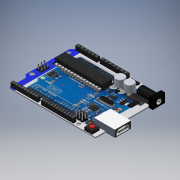
# Autodesk Inventor part: ardino
Saved by Autodesk Inventor 2019 (Build 230136000, 136)
## iProperties
Created: 2020-12-08
Part Number: ardino
Material: Aluminum 6061-AHC
Document SubType Name: Modeling
Designer: 2019u
Density: 2.7 g/cm^3
Appearance: Aluminum - Polished
Author: 2019u
Autodesk Inventor part; units mm, degrees
ref_plane "YZ Plane" through (0, 0, 0) normal (1, 0, 0) x (0, 1, 0)
ref_plane "XZ Plane" through (0, 0, 0) normal (0, 1, 0) x (-1, 0, 0)
ref_plane "XY Plane" through (0, 0, 0) normal (0, 0, 1) x (1, 0, 0)
sketch "Sketch1" plane through (0, 0, 0) normal (0, 1, 0) x (-1, 0, 0)
  line L0 (0, 0) -> (99.3908, 0) construction
  line L1 (99.3908, 0) -> (99.3908, -99.3908) construction
  line L2 (99.3908, -99.3908) -> (0, -99.3908) construction
  line L3 (0, -99.3908) -> (0, 0) construction
  line L4 (94.1362, -15.3552) -> (10.2114, -15.3552)
  line L5 (10.2114, -15.3552) -> (10.2114, -25.1728)
  line L6 (10.2114, -25.1728) -> (0, -25.1728)
  line L7 (1.1362, -25.1728) -> (1.1362, -40.953)
  line L8 (1.1362, -40.953) -> (10.2114, -40.953)
  line L9 (10.2114, -40.953) -> (10.2114, -67.1342)
  line L10 (10.2114, -67.1342) -> (8.5885, -67.1342)
  line L11 (6.3655, -68.1381) -> (6.3655, -79.1042)
  line L12 (8.5885, -79.5442) -> (10.2114, -79.5442)
  line L13 (10.2114, -79.5442) -> (10.2114, -83.1265)
  line L14 (10.2114, -83.1265) -> (94.9443, -83.1265)
  line L15 (94.9443, -83.1265) -> (94.9443, -80.9195)
  line L16 (94.9443, -80.9195) -> (97.9355, -77.6084)
  line L17 (97.9355, -77.6084) -> (98.096, -34.4505)
  line L18 (98.096, -34.4505) -> (94.9443, -31.6032)
  line L19 (94.9443, -31.6032) -> (95.0011, -16.3408)
  arc A0 (95.0011, -16.3408) -> (94.1362, -15.3552) centre (93.5899, -16.7068) ccw
  line L20 (10.2114, -25.1728) -> (21.2581, -25.1728)
  line L21 (21.2581, -25.1728) -> (21.2581, -40.953)
  line L22 (21.2581, -40.953) -> (10.2114, -40.953)
  line L23 (10.2114, -67.1342) -> (10.2114, -68.0566)
  line L24 (10.2114, -79.1042) -> (10.2114, -79.5442)
  line L25 (94.5949, -16.4252) -> (68.0366, -16.4252)
  line L26 (68.0366, -16.4252) -> (68.0366, -19.2086)
  line L27 (68.0366, -19.2086) -> (94.5949, -19.2086)
  line L28 (94.5949, -19.2086) -> (94.5949, -16.4252)
  line L29 (64.6828, -16.0728) -> (32.7155, -16.0728)
  line L30 (32.7155, -16.0728) -> (32.7155, -18.833)
  line L31 (32.7155, -18.833) -> (64.6828, -18.833)
  line L32 (64.6828, -18.833) -> (64.6828, -16.0728)
  line L33 (92.7813, -58.1151) -> (46.6733, -58.1151)
  line L34 (46.6733, -58.1151) -> (46.6733, -67.7931)
  line L35 (46.6733, -67.7931) -> (92.7813, -67.7931)
  line L36 (92.7813, -67.7931) -> (92.7813, -58.1151)
  line L37 (38.3786, -36.2645) -> (32.5411, -36.2645)
  line L38 (32.5411, -36.2645) -> (32.5411, -41.7109)
  line L39 (32.5411, -41.7109) -> (38.3786, -41.7109)
  line L40 (38.3786, -41.7109) -> (38.3786, -36.2645)
  line L41 (38.0929, -47.7922) -> (29.7352, -47.7922)
  line L42 (29.7352, -47.7922) -> (29.7352, -52.5671)
  line L43 (29.7352, -52.5671) -> (38.0929, -52.5671)
  line L44 (38.0929, -52.5671) -> (38.0929, -47.7922)
  arc A1 (38.0929, -52.5671) -> (38.0929, -47.7922) centre (38.0929, -50.1797) ccw
  arc A2 (29.7352, -47.7922) -> (29.7352, -52.5671) centre (29.7352, -50.1797) ccw
  circle A3 centre (42.8477, -72.0836) radius 4.3989
  circle A4 centre (33.5477, -72.0836) radius 4.3076
  line L45 (36.2266, -55.7996) -> (32.5411, -55.7996)
  line L46 (32.5411, -55.7996) -> (32.5411, -59.4796)
  line L47 (32.5411, -59.4796) -> (36.2266, -59.4796)
  line L48 (36.2266, -59.4796) -> (36.2266, -55.7996)
  line L49 (94.1362, -79.3242) -> (72.919, -79.3242)
  line L50 (72.919, -79.3242) -> (72.919, -82.3228)
  line L51 (72.919, -82.3228) -> (94.1362, -82.3228)
  line L52 (94.1362, -82.3228) -> (94.1362, -79.3242)
  line L53 (70.678, -79.9168) -> (44.0674, -79.9168)
  line L54 (44.0674, -79.9168) -> (44.0674, -82.6646)
  line L55 (44.0674, -82.6646) -> (70.678, -82.6646)
  line L56 (70.678, -82.6646) -> (70.678, -79.9168)
  line L57 (41.6475, -79.3242) -> (33.5477, -79.3242)
  line L58 (33.5477, -79.3242) -> (33.5477, -82.3228)
  line L59 (33.5477, -82.3228) -> (41.6475, -82.3228)
  line L60 (41.6475, -82.3228) -> (41.6475, -79.3242)
  line L61 (91.1629, -43.127) -> (96.9206, -43.127)
  line L62 (96.9206, -43.127) -> (96.9206, -52.2064)
  line L63 (96.9206, -52.2064) -> (91.1629, -52.2064)
  line L64 (91.1629, -52.2064) -> (91.1629, -43.127)
  line L65 (10.2114, -68.0566) -> (10.2114, -79.1042)
  line L66 (10.2114, -78.709) -> (10.2114, -67.1342)
  line L67 (10.2114, -79.1042) -> (10.2114, -79.5442)
  line L68 (10.2114, -79.5442) -> (6.3655, -79.5442)
  line L69 (6.3655, -79.5442) -> (6.3655, -67.5295)
  line L70 (6.3655, -67.5295) -> (10.2114, -67.5295)
  line L71 (10.2114, -67.5295) -> (10.2114, -79.5442)
  line L72 (10.2114, -78.0442) -> (24.0286, -78.0442)
  line L73 (24.0286, -78.0442) -> (24.0286, -69.0295)
  line L74 (24.0286, -69.0295) -> (10.2114, -69.0295)
  line L75 (10.2114, -69.0295) -> (10.2114, -78.0442)
  circle A5 centre (17.5453, -19.2086) radius 2.0145
  line L76 (14.0816, -23.069) -> (21.6028, -23.069)
  line L77 (21.6028, -23.069) -> (21.6028, -15.7452)
  line L78 (21.6028, -15.7452) -> (14.0816, -15.7452)
  line L79 (14.0816, -15.7452) -> (14.0816, -23.069)
  line L80 (28.7929, -26.9178) -> (37.8553, -26.9178)
  line L81 (37.8553, -26.9178) -> (37.8553, -20.8454)
  line L82 (37.8553, -20.8454) -> (28.7929, -20.8454)
  line L83 (28.7929, -20.8454) -> (28.7929, -26.9178)
  line L84 (29.24, -26.4718) -> (31.1601, -26.4718)
  line L85 (31.1601, -26.4718) -> (31.1601, -24.2418)
  line L86 (31.1601, -24.2418) -> (29.24, -24.2418)
  line L87 (29.24, -24.2418) -> (29.24, -26.4718)
  line L88 (32.24, -24.2418) -> (32.24, -26.4718)
  line L89 (34.1601, -26.4718) -> (34.1601, -24.2418)
  line L90 (32.24, -26.4718) -> (34.1601, -26.4718)
  line L91 (34.1601, -24.2418) -> (32.24, -24.2418)
  line L92 (35.24, -24.2418) -> (35.24, -26.4718)
  line L93 (37.1601, -26.4718) -> (37.1601, -24.2418)
  line L94 (35.24, -26.4718) -> (37.1601, -26.4718)
  line L95 (37.1601, -24.2418) -> (35.24, -24.2418)
  line L96 (29.24, -21.2418) -> (29.24, -23.4718)
  line L97 (31.1601, -23.4718) -> (31.1601, -21.2418)
  line L98 (29.24, -23.4718) -> (31.1601, -23.4718)
  line L99 (31.1601, -21.2418) -> (29.24, -21.2418)
  line L100 (32.24, -21.2418) -> (32.24, -23.4718)
  line L101 (34.1601, -23.4718) -> (34.1601, -21.2418)
  line L102 (32.24, -23.4718) -> (34.1601, -23.4718)
  line L103 (34.1601, -21.2418) -> (32.24, -21.2418)
  line L104 (35.24, -21.2418) -> (35.24, -23.4718)
  line L105 (37.1601, -23.4718) -> (37.1601, -21.2418)
  line L106 (35.24, -23.4718) -> (37.1601, -23.4718)
  line L107 (37.1601, -21.2418) -> (35.24, -21.2418)
  circle A6 centre (30.2001, -25.3568) radius 0.4649
  circle A7 centre (33.2001, -25.3568) radius 0.4846
  circle A8 centre (36.2001, -25.3568) radius 0.4567
  circle A9 centre (30.119, -22.3568) radius 0.4825
  circle A10 centre (33.2001, -22.3568) radius 0.4846
  circle A11 centre (36.2001, -22.3568) radius 0.4846
  line L108 (91.1629, -49.1995) -> (100.2253, -49.1995)
  line L109 (100.2253, -49.1995) -> (100.2253, -43.127)
  line L110 (100.2253, -43.127) -> (91.1629, -43.127)
  line L111 (91.1629, -43.127) -> (91.1629, -49.1995)
  line L112 (91.61, -48.7535) -> (93.5302, -48.7535)
  line L113 (93.5302, -48.7535) -> (93.5302, -46.5235)
  line L114 (93.5302, -46.5235) -> (91.61, -46.5235)
  line L115 (91.61, -46.5235) -> (91.61, -48.7535)
  line L116 (94.61, -46.5235) -> (94.61, -48.7535)
  line L117 (96.5302, -48.7535) -> (96.5302, -46.5235)
  line L118 (94.61, -48.7535) -> (96.5302, -48.7535)
  line L119 (96.5302, -46.5235) -> (94.61, -46.5235)
  line L120 (97.61, -46.5235) -> (97.61, -48.7535)
  line L121 (99.5302, -48.7535) -> (99.5302, -46.5235)
  line L122 (97.61, -48.7535) -> (99.5302, -48.7535)
  line L123 (99.5302, -46.5235) -> (97.61, -46.5235)
  line L124 (91.61, -43.5235) -> (91.61, -45.7535)
  line L125 (93.5302, -45.7535) -> (93.5302, -43.5235)
  line L126 (91.61, -45.7535) -> (93.5302, -45.7535)
  line L127 (93.5302, -43.5235) -> (91.61, -43.5235)
  line L128 (94.61, -43.5235) -> (94.61, -45.7535)
  line L129 (96.5302, -45.7535) -> (96.5302, -43.5235)
  line L130 (94.61, -45.7535) -> (96.5302, -45.7535)
  line L131 (96.5302, -43.5235) -> (94.61, -43.5235)
  line L132 (97.61, -43.5235) -> (97.61, -45.7535)
  line L133 (99.5302, -45.7535) -> (99.5302, -43.5235)
  line L134 (97.61, -45.7535) -> (99.5302, -45.7535)
  line L135 (99.5302, -43.5235) -> (97.61, -43.5235)
  circle A12 centre (92.5701, -47.6385) radius 0.4649
  circle A13 centre (95.5701, -47.6385) radius 0.4846
  circle A14 centre (98.5701, -47.6385) radius 0.4567
  circle A15 centre (92.489, -44.6385) radius 0.4825
  circle A16 centre (95.5701, -44.6385) radius 0.4846
  circle A17 centre (98.5701, -44.6385) radius 0.4846
  line L136 (94.61, -51.6653) -> (96.5302, -51.6653)
  circle A18 centre (95.5701, -50.5503) radius 0.4846
  line L137 (94.61, -49.4353) -> (94.61, -51.6653)
  line L138 (96.5302, -51.6653) -> (96.5302, -49.4353)
  line L139 (96.5302, -49.4353) -> (94.61, -49.4353)
  line L140 (97.61, -49.4353) -> (97.61, -51.6653)
  line L141 (91.61, -51.6653) -> (93.5302, -51.6653)
  circle A19 centre (92.5701, -50.5503) radius 0.4649
  line L142 (91.61, -49.4353) -> (91.61, -51.6653)
  line L143 (93.5302, -51.6653) -> (93.5302, -49.4353)
  line L144 (93.5302, -49.4353) -> (91.61, -49.4353)
  line L145 (17.5453, -65.908) -> (21.2581, -65.908)
  line L146 (21.2581, -65.908) -> (21.2581, -57.6396)
  line L147 (21.2581, -57.6396) -> (17.5453, -57.6396)
  line L148 (17.5453, -57.6396) -> (17.5453, -65.908)
  line L149 (37.1601, -66.1422) -> (38.7457, -66.1422)
  line L150 (38.7457, -66.1422) -> (38.7457, -62.7647)
  line L151 (38.7457, -62.7647) -> (37.1601, -62.7647)
  line L152 (37.1601, -62.7647) -> (37.1601, -66.1422)
  line L153 (47.2465, -58.1151) -> (49.4015, -58.1151)
  line L154 (49.4015, -58.1151) -> (49.4015, -56.2579)
  line L155 (49.4015, -56.2579) -> (47.2465, -56.2579)
  line L156 (47.2465, -56.2579) -> (47.2465, -58.1151)
  line L157 (50.2465, -56.2579) -> (50.2465, -58.1151)
  line L158 (52.4015, -56.2579) -> (50.2465, -56.2579)
  line L159 (52.4015, -58.1151) -> (52.4015, -56.2579)
  line L160 (50.2465, -58.1151) -> (52.4015, -58.1151)
  line L161 (53.2465, -56.2579) -> (53.2465, -58.1151)
  line L162 (55.4015, -56.2579) -> (53.2465, -56.2579)
  line L163 (55.4015, -58.1151) -> (55.4015, -56.2579)
  line L164 (53.2465, -58.1151) -> (55.4015, -58.1151)
  line L165 (56.2465, -56.2579) -> (56.2465, -58.1151)
  line L166 (58.4015, -56.2579) -> (56.2465, -56.2579)
  line L167 (58.4015, -58.1151) -> (58.4015, -56.2579)
  line L168 (56.2465, -58.1151) -> (58.4015, -58.1151)
  line L169 (59.2465, -56.2579) -> (59.2465, -58.1151)
  line L170 (61.4015, -56.2579) -> (59.2465, -56.2579)
  line L171 (61.4015, -58.1151) -> (61.4015, -56.2579)
  line L172 (59.2465, -58.1151) -> (61.4015, -58.1151)
  line L173 (62.2465, -56.2579) -> (62.2465, -58.1151)
  line L174 (64.4015, -56.2579) -> (62.2465, -56.2579)
  line L175 (64.4015, -58.1151) -> (64.4015, -56.2579)
  line L176 (62.2465, -58.1151) -> (64.4015, -58.1151)
  line L177 (65.2465, -56.2579) -> (65.2465, -58.1151)
  line L178 (67.4015, -56.2579) -> (65.2465, -56.2579)
  line L179 (67.4015, -58.1151) -> (67.4015, -56.2579)
  line L180 (65.2465, -58.1151) -> (67.4015, -58.1151)
  line L181 (68.2465, -56.2579) -> (68.2465, -58.1151)
  line L182 (70.4015, -56.2579) -> (68.2465, -56.2579)
  line L183 (70.4015, -58.1151) -> (70.4015, -56.2579)
  line L184 (68.2465, -58.1151) -> (70.4015, -58.1151)
  line L185 (71.2465, -56.2579) -> (71.2465, -58.1151)
  line L186 (73.4015, -56.2579) -> (71.2465, -56.2579)
  line L187 (73.4015, -58.1151) -> (73.4015, -56.2579)
  line L188 (71.2465, -58.1151) -> (73.4015, -58.1151)
  line L189 (74.2465, -56.2579) -> (74.2465, -58.1151)
  line L190 (76.4015, -56.2579) -> (74.2465, -56.2579)
  line L191 (76.4015, -58.1151) -> (76.4015, -56.2579)
  line L192 (74.2465, -58.1151) -> (76.4015, -58.1151)
  line L193 (77.2465, -56.2579) -> (77.2465, -58.1151)
  line L194 (79.4015, -56.2579) -> (77.2465, -56.2579)
  line L195 (79.4015, -58.1151) -> (79.4015, -56.2579)
  line L196 (77.2465, -58.1151) -> (79.4015, -58.1151)
  line L197 (80.2465, -56.2579) -> (80.2465, -58.1151)
  line L198 (82.4015, -56.2579) -> (80.2465, -56.2579)
  line L199 (82.4015, -58.1151) -> (82.4015, -56.2579)
  line L200 (80.2465, -58.1151) -> (82.4015, -58.1151)
  line L201 (83.2465, -56.2579) -> (83.2465, -58.1151)
  line L202 (85.4015, -56.2579) -> (83.2465, -56.2579)
  line L203 (85.4015, -58.1151) -> (85.4015, -56.2579)
  line L204 (83.2465, -58.1151) -> (85.4015, -58.1151)
  line L205 (86.2465, -56.2579) -> (86.2465, -58.1151)
  line L206 (88.4015, -56.2579) -> (86.2465, -56.2579)
  line L207 (88.4015, -58.1151) -> (88.4015, -56.2579)
  line L208 (86.2465, -58.1151) -> (88.4015, -58.1151)
  line L209 (89.2465, -56.2579) -> (89.2465, -58.1151)
  line L210 (91.4015, -56.2579) -> (89.2465, -56.2579)
  line L211 (91.4015, -58.1151) -> (91.4015, -56.2579)
  line L212 (89.2465, -58.1151) -> (91.4015, -58.1151)
  line L213 (47.2465, -67.7747) -> (47.2465, -69.6318)
  line L214 (49.4015, -67.7747) -> (47.2465, -67.7747)
  line L215 (49.4015, -69.6318) -> (49.4015, -67.7747)
  line L216 (47.2465, -69.6318) -> (49.4015, -69.6318)
  line L217 (50.2465, -67.7747) -> (50.2465, -69.6318)
  line L218 (52.4015, -67.7747) -> (50.2465, -67.7747)
  line L219 (52.4015, -69.6318) -> (52.4015, -67.7747)
  line L220 (50.2465, -69.6318) -> (52.4015, -69.6318)
  line L221 (53.2465, -67.7747) -> (53.2465, -69.6318)
  line L222 (55.4015, -67.7747) -> (53.2465, -67.7747)
  line L223 (55.4015, -69.6318) -> (55.4015, -67.7747)
  line L224 (53.2465, -69.6318) -> (55.4015, -69.6318)
  line L225 (56.2465, -67.7747) -> (56.2465, -69.6318)
  line L226 (58.4015, -67.7747) -> (56.2465, -67.7747)
  line L227 (58.4015, -69.6318) -> (58.4015, -67.7747)
  line L228 (56.2465, -69.6318) -> (58.4015, -69.6318)
  line L229 (59.2465, -67.7747) -> (59.2465, -69.6318)
  line L230 (61.4015, -67.7747) -> (59.2465, -67.7747)
  line L231 (61.4015, -69.6318) -> (61.4015, -67.7747)
  line L232 (59.2465, -69.6318) -> (61.4015, -69.6318)
  line L233 (62.2465, -67.7747) -> (62.2465, -69.6318)
  line L234 (64.4015, -67.7747) -> (62.2465, -67.7747)
  line L235 (64.4015, -69.6318) -> (64.4015, -67.7747)
  line L236 (62.2465, -69.6318) -> (64.4015, -69.6318)
  line L237 (65.2465, -67.7747) -> (65.2465, -69.6318)
  line L238 (67.4015, -67.7747) -> (65.2465, -67.7747)
  line L239 (67.4015, -69.6318) -> (67.4015, -67.7747)
  line L240 (65.2465, -69.6318) -> (67.4015, -69.6318)
  line L241 (68.2465, -67.7747) -> (68.2465, -69.6318)
  line L242 (70.4015, -67.7747) -> (68.2465, -67.7747)
  line L243 (70.4015, -69.6318) -> (70.4015, -67.7747)
  line L244 (68.2465, -69.6318) -> (70.4015, -69.6318)
  line L245 (71.2465, -67.7747) -> (71.2465, -69.6318)
  line L246 (73.4015, -67.7747) -> (71.2465, -67.7747)
  line L247 (73.4015, -69.6318) -> (73.4015, -67.7747)
  line L248 (71.2465, -69.6318) -> (73.4015, -69.6318)
  line L249 (74.2465, -67.7747) -> (74.2465, -69.6318)
  line L250 (76.4015, -67.7747) -> (74.2465, -67.7747)
  line L251 (76.4015, -69.6318) -> (76.4015, -67.7747)
  line L252 (74.2465, -69.6318) -> (76.4015, -69.6318)
  line L253 (77.2465, -67.7747) -> (77.2465, -69.6318)
  line L254 (79.4015, -67.7747) -> (77.2465, -67.7747)
  line L255 (79.4015, -69.6318) -> (79.4015, -67.7747)
  line L256 (77.2465, -69.6318) -> (79.4015, -69.6318)
  line L257 (80.2465, -67.7747) -> (80.2465, -69.6318)
  line L258 (82.4015, -67.7747) -> (80.2465, -67.7747)
  line L259 (82.4015, -69.6318) -> (82.4015, -67.7747)
  line L260 (80.2465, -69.6318) -> (82.4015, -69.6318)
  line L261 (83.2465, -67.7747) -> (83.2465, -69.6318)
  line L262 (85.4015, -67.7747) -> (83.2465, -67.7747)
  line L263 (85.4015, -69.6318) -> (85.4015, -67.7747)
  line L264 (83.2465, -69.6318) -> (85.4015, -69.6318)
  line L265 (86.2465, -67.7747) -> (86.2465, -69.6318)
  line L266 (88.4015, -67.7747) -> (86.2465, -67.7747)
  line L267 (88.4015, -69.6318) -> (88.4015, -67.7747)
  line L268 (86.2465, -69.6318) -> (88.4015, -69.6318)
  line L269 (89.2465, -67.7747) -> (89.2465, -69.6318)
  line L270 (91.4015, -67.7747) -> (89.2465, -67.7747)
  line L271 (91.4015, -69.6318) -> (91.4015, -67.7747)
  line L272 (89.2465, -69.6318) -> (91.4015, -69.6318)
  line L273 (93.5302, -56.2579) -> (46.4999, -56.2579)
  line L274 (46.4999, -56.2579) -> (46.4999, -69.6318)
  line L275 (46.4999, -69.6318) -> (93.5302, -69.6318)
  line L276 (93.5302, -69.6318) -> (93.5302, -56.2579)
  dimension "d4" = 9.3
  dimension "d68" = 1.5
  dimension "d69" = 1.5
  dimension "d83" = 3
  dimension "d86" = 3
  dimension "d99" = 3
  dimension "d100" = 3
  dimension "d112" = 3
  dimension "d133" = 3
  dimension "d136" = 11.5168
  dimension "d194" = 99.3908
  constraints: 546 end point, 46 parallel, 32 perpendicular, 27 horizontal, 19 centre point, 12 point on line, 6 point on circle, 5 vertical, 4 tangent, 317 other
  measures "d4" distance of A4.centre point (42.848, -72.084)
  measures "d68" distance between parallel lines of L74 L70
  measures "d69" distance between parallel lines of L72 L68
  measures "d83" distance of L86.end L88.start
  measures "d86" distance of L86.end L96.start
  measures "d99" distance of L115.start L116.start
  measures "d100" distance of L115.start L124.start
  measures "d112" distance of L144.end L139.end
  measures "d133" distance of L155.end L157.start
  measures "d136" distance of L155.end L213.start
  measures "d194" distance of L2.end L1.end
extrude "Extrusion1" add sketch "Sketch1" against normal blind 1 contours A0 L19 L18 L17 L110 L61 L64 L63 L62 L108 L16 L15 L14 L13 L24 L65 L72 L73 L74 L23 L9 L22 L21 L20 L5 L4 | L17 L135 L132 L134 L123 L120 L122 L108 L62 L110 | L17 L134 L132 L135 | L62 L108 L64 L61 | L62 L63 L64 L108 | L17 L122 L120 L123 | L74 L73 L72 L65 | L28 L27 L26 L25 | L32 L31 L30 L29 | L36 L35 L271 L270 L269 L267 L266 L265 L263 L262 L261 L259 L258 L257 L255 L254 L253 L251 L250 L249 L247 L246 L245 L243 L242 L241 L239 L238 L237 L235 L234 L233 L231 L230 L229 L227 L226 L225 L223 L222 L221 L219 L218 L217 L215 L214 L213 L34 L33 | L33 L211 L273 L276 L275 L271 L35 L36 | L33 L209 L210 L211 | L33 L207 L273 L209 | A3 | L271 L272 L269 L35 | L35 L269 L270 L271 | L33 L205 L206 L207 | L269 L275 L267 L35 | L33 L203 L273 L205 | L267 L268 L265 L35 | L35 L265 L266 L267 | L33 L201 L202 L203 | L265 L275 L263 L35 | L33 L199 L273 L201 | L263 L264 L261 L35 | L35 L261 L262 L263 | L33 L197 L198 L199 | L261 L275 L259 L35 | L33 L195 L273 L197 | L259 L260 L257 L35 | L35 L257 L258 L259 | L33 L193 L194 L195 | L257 L275 L255 L35 | L33 L191 L273 L193 | L255 L256 L253 L35 | L35 L253 L254 L255 | L33 L189 L190 L191 | L253 L275 L251 L35 | L33 L187 L273 L189 | L251 L252 L249 L35 | L35 L249 L250 L251 | L33 L185 L186 L187 | L249 L275 L247 L35 | L33 L183 L273 L185 | L247 L248 L245 L35 | L35 L245 L246 L247 | L33 L181 L182 L183 | L245 L275 L243 L35 | L33 L179 L273 L181 | L243 L244 L241 L35 | L35 L241 L242 L243 | L33 L177 L178 L179 | L241 L275 L239 L35 | L33 L175 L273 L177 | L239 L240 L237 L35 | L35 L237 L238 L239 | L33 L173 L174 L175 | L237 L275 L235 L35 | L33 L171 L273 L173 | L235 L236 L233 L35 | L35 L233 L234 L235 | L33 L169 L170 L171 | L233 L275 L231 L35 | L33 L167 L273 L169 | L231 L232 L229 L35 | L35 L229 L230 L231 | L33 L165 L166 L167 | L229 L275 L227 L35 | L33 L163 L273 L165 | L227 L228 L225 L35 | L35 L225 L226 L227 | L33 L161 L162 L163 | L225 L275 L223 L35 | L33 L159 L273 L161 | L223 L224 L221 L35 | L35 L221 L222 L223 | L33 L157 L158 L159 | L221 L275 L219 L35 | L33 L154 L273 L157 | L219 L220 L217 L35 | L35 L217 L218 L219 | L33 L156 L155 L154 | L217 L275 L215 L35 | L33 L34 L35 L213 L275 L274 L273 L156 | L215 L216 L213 L35 | L35 L213 L214 L215 | L40 L39 L38 L37 | L44 L43 L42 L41 | A1 L44 | L42 A2 | A4 | L48 L47 L46 L45 | L52 L51 L50 L49 | L56 L55 L54 L53 | L60 L59 L58 L57 | A5 | L79 L78 L77 L76 | L83 L82 L81 L80 | L87 L86 L85 L84 | L91 L89 L90 L88 | L95 L93 L94 L92 | L99 L97 L98 L96 | L103 L101 L102 L100 | L107 L105 L106 L104 | A6 | A7 | A8 | A9 | A10 | A11 | L115 L114 L113 L112 | L119 L117 L118 L116 | L127 L125 L126 L124 | L131 L129 L130 L128 | A12 | A13 | A15 | A16 | L137 L139 L138 L136 | A18 | L142 L144 L143 L141 | A19 | L148 L147 L146 L145 | L152 L151 L150 L149
extrude "Extrusion2" add sketch "Sketch1" along normal blind 6 and the other way blind 1 contours L20 L21 L22 L8 L7 L6
extrude "Extrusion3" add sketch "Sketch1" along normal blind 7 contours A3 | A4
extrude "Extrusion4" add sketch "Sketch1" along normal blind 5 contours L36 L35 L271 L270 L269 L267 L266 L265 L263 L262 L261 L259 L258 L257 L255 L254 L253 L251 L250 L249 L247 L246 L245 L243 L242 L241 L239 L238 L237 L235 L234 L233 L231 L230 L229 L227 L226 L225 L223 L222 L221 L219 L218 L217 L215 L214 L213 L34 L33 | L35 L269 L270 L271 | L35 L265 L266 L267 | L35 L261 L262 L263 | L35 L257 L258 L259 | L35 L253 L254 L255 | L35 L249 L250 L251 | L35 L245 L246 L247 | L35 L241 L242 L243 | L35 L237 L238 L239 | L35 L233 L234 L235 | L35 L229 L230 L231 | L35 L225 L226 L227 | L35 L221 L222 L223 | L35 L217 L218 L219 | L35 L213 L214 L215
extrude "Extrusion5" add sketch "Sketch1" along normal blind 2 contours L44 L43 L42 L41 | A1 L44 | L42 A2
extrude "Extrusion6" add sketch "Sketch1" along normal blind 0.5 contours L40 L39 L38 L37 | L48 L47 L46 L45
extrude "Extrusion7" add sketch "Sketch1" along normal blind 4 contours L28 L27 L26 L25 | L32 L31 L30 L29 | L52 L51 L50 L49 | L56 L55 L54 L53
extrude "Extrusion10" add sketch "Sketch1" along normal blind 8 and the other way blind 1 contours L23 L65 L24 L12 L68 L69 L11 L70
extrude "Extrusion11" add sketch "Sketch1" along normal blind 8 contours L74 L73 L72 L65
fillet "Fillet2" radius 4.5 2 edges at (-17.12, 8, -78.0442) (-17.12, 8, -69.0295)
extrude "Extrusion12" add sketch "Sketch1" along normal blind 4 contours A5
extrude "Extrusion13" add sketch "Sketch1" along normal blind 3 contours L79 L78 L77 L76
extrude "Extrusion14" add sketch "Sketch1" along normal blind 5 contours A6 | A7 | A8 | A9 | A10 | A11
extrude "Extrusion15" add sketch "Sketch1" along normal blind 1 contours L87 L86 L85 L84 | L91 L89 L90 L88 | L95 L93 L94 L92 | L99 L97 L98 L96 | L103 L101 L102 L100 | L107 L105 L106 L104
fillet "Fillet3" radius 0.4 6 edges at (-29.7352, 5, -25.3568) (-29.6365, 5, -22.3568) (-32.7155, 5, -25.3568) (-35.7434, 5, -25.3568) (-35.7155, 5, -22.3568) (-32.7155, 5, -22.3568)
extrude "Extrusion16" add sketch "Sketch1" along normal blind 5 contours A12 | A13 | A15 | A16 | A18 | A19
extrude "Extrusion17" add sketch "Sketch1" along normal blind 1 contours L115 L114 L113 L112 | L119 L117 L118 L116 | L127 L125 L126 L124 | L131 L129 L130 L128 | L137 L139 L138 L136 | L142 L144 L143 L141
fillet "Fillet4" radius 0.4 30 edges at (-92.0065, 5, -44.6385) (-95.0855, 5, -44.6385) (-92.1052, 5, -47.6385) (-91.61, 1, -47.6385) (-95.0855, 5, -47.6385) (-95.0855, 5, -50.5503) (-92.1052, 5, -50.5503) (-92.5701, 1, -48.7535) (-93.5302, 1, -47.6385) (-92.5701, 1, -46.5235) (-91.61, 1, -44.6385) (-92.5701, 1, -45.7535) (-92.5701, 1, -43.5235) (-93.5302, 1, -44.6385) (-94.61, 1, -44.6385) (-95.5701, 1, -43.5235) (-96.5302, 1, -44.6385) (-95.5701, 1, -45.7535) (-95.5701, 1, -46.5235) (-94.61, 1, -47.6385) (-95.5701, 1, -48.7535) (-96.5302, 1, -47.6385) (-91.61, 1, -50.5503) (-92.5701, 1, -51.6653) (-92.5701, 1, -49.4353) (-93.5302, 1, -50.5503) (-94.61, 1, -50.5503) (-95.5701, 1, -51.6653) (-95.5701, 1, -49.4353) (-96.5302, 1, -50.5503)
extrude "Extrusion18" add sketch "Sketch1" along normal blind 1 contours L60 L59 L58 L57
extrude "Extrusion19" add sketch "Sketch1" along normal blind 1 contours L148 L147 L146 L145 | L152 L151 L150 L149
sketch "Sketch2" plane through (-6.3655, -1, -79.5442) normal (1, 0, 0) x (0, 0, -1)
  circle A0 centre (-5.7758, 4.0263) radius 2.4717
  circle A1 centre (-5.7758, 4.0263) radius 0.5901
  point P0 (-79.5442, 1)
  constraints: 2 centre point, 1 coincident
extrude "Extrusion20" cut sketch "Sketch2" against normal blind 15
sketch "Sketch3" plane through (-1.1362, -1, -40.953) normal (1, 0, 0) x (0, 0, -1)
  line L0 (-11.132, 5.6691) -> (-4.7121, 5.6691)
  line L1 (-1.7121, 2.6691) -> (-1.7121, 0.6321)
  line L2 (-1.7121, 0.6321) -> (-14.132, 0.6321)
  line L3 (-14.132, 0.6321) -> (-14.132, 2.6691)
  arc A0 (-11.132, 5.6691) -> (-14.132, 2.6691) centre (-11.132, 2.6691) ccw
  arc A1 (-1.7121, 2.6691) -> (-4.7121, 5.6691) centre (-4.7121, 2.6691) ccw
  line L4 (-4.7121, 3.9211) -> (-11.132, 3.9211)
  arc A2 (-11.132, 3.9211) -> (-12.384, 2.6691) centre (-11.132, 2.6691) ccw
  line L5 (-12.384, 2.6691) -> (-12.384, 2.3801)
  line L6 (-12.384, 2.3801) -> (-3.4601, 2.3801)
  line L7 (-3.4601, 2.3801) -> (-3.4601, 2.6691)
  arc A3 (-3.4601, 2.6691) -> (-4.7121, 3.9211) centre (-4.7121, 2.6691) ccw
  line L8 (-10.6435, 3.3982) -> (-5.0624, 3.3982)
  line L9 (-5.0624, 3.3982) -> (-5.0624, 2.8158)
  line L10 (-5.0624, 2.8158) -> (-10.6435, 2.8158)
  line L11 (-10.6435, 2.8158) -> (-10.6435, 3.3982)
  line L12 (-10.6435, 2.8158) -> (-10.2916, 2.8158)
  line L13 (-10.2916, 2.8158) -> (-10.2916, 3.107)
  line L14 (-10.2916, 3.107) -> (-10.6435, 3.107)
  line L15 (-10.6435, 3.107) -> (-10.6435, 2.8158)
  line L16 (-9.8886, 2.8158) -> (-9.5394, 2.8158)
  line L17 (-9.5394, 2.8158) -> (-9.5394, 3.107)
  line L18 (-9.5394, 3.107) -> (-9.8886, 3.107)
  line L19 (-9.8886, 3.107) -> (-9.8886, 2.8158)
  line L20 (-9.1148, 3.107) -> (-8.6537, 3.107)
  line L21 (-8.6537, 3.107) -> (-8.6537, 2.8158)
  line L22 (-8.6537, 2.8158) -> (-9.1148, 2.8158)
  line L23 (-9.1148, 2.8158) -> (-9.1148, 3.107)
  line L24 (-8.3261, 3.107) -> (-8.0592, 3.107)
  line L25 (-8.0592, 3.107) -> (-8.0592, 2.8158)
  line L26 (-8.0592, 2.8158) -> (-8.3261, 2.8158)
  line L27 (-8.3261, 2.8158) -> (-8.3261, 3.107)
  line L28 (-7.853, 3.107) -> (-7.7085, 3.107)
  line L29 (-7.7085, 3.107) -> (-7.7085, 2.8158)
  line L30 (-7.7085, 2.8158) -> (-7.853, 2.8158)
  line L31 (-7.853, 2.8158) -> (-7.853, 3.107)
  line L32 (-7.4162, 3.107) -> (-7.1735, 3.107)
  line L33 (-7.1735, 3.107) -> (-7.1735, 2.8158)
  line L34 (-7.1735, 2.8158) -> (-7.4162, 2.8158)
  line L35 (-7.4162, 2.8158) -> (-7.4162, 3.107)
  line L36 (-6.8945, 3.107) -> (-6.6397, 3.107)
  line L37 (-6.6397, 3.107) -> (-6.6397, 2.8158)
  line L38 (-6.6397, 2.8158) -> (-6.8945, 2.8158)
  line L39 (-6.8945, 2.8158) -> (-6.8945, 3.107)
  line L40 (-6.3485, 3.107) -> (-6.0937, 3.107)
  line L41 (-6.0937, 3.107) -> (-6.0937, 2.8158)
  line L42 (-6.0937, 2.8158) -> (-6.3485, 2.8158)
  line L43 (-6.3485, 2.8158) -> (-6.3485, 3.107)
  line L44 (-5.8025, 3.107) -> (-5.5841, 3.107)
  line L45 (-5.5841, 3.107) -> (-5.5841, 2.8158)
  line L46 (-5.5841, 2.8158) -> (-5.8025, 2.8158)
  line L47 (-5.8025, 2.8158) -> (-5.8025, 3.107)
  line L48 (-5.39, 3.107) -> (-5.2444, 3.107)
  line L49 (-5.2444, 3.107) -> (-5.2444, 2.8158)
  line L50 (-5.2444, 2.8158) -> (-5.39, 2.8158)
  line L51 (-5.39, 2.8158) -> (-5.39, 3.107)
  point P0 (-40.953, 1)
  dimension "d128" = 3
  constraints: 102 end point, 25 parallel, 13 horizontal, 13 perpendicular, 9 point on line, 8 point on circle, 4 centre point, 4 tangent, 1 equal radius, 17 other
  measures "d128" radius of A0
extrude "Extrusion21" cut sketch "Sketch3" against normal blind 15 contours L0 A1 L1 L2 L3 A0 | L8 L9 L10 L49 L48 L51 L45 L44 L47 L41 L40 L43 L37 L36 L39 L33 L32 L35 L29 L28 L31 L25 L24 L27 L21 L20 L23 L17 L18 L19 L13 L14 L11
extrude "Extrusion22" add sketch "Sketch1" along normal blind 1.5 contours L33 L156 L155 L154
pattern_linear "Rectangular Pattern1" count 15 spacing 3 along (-1, 0, 0) count 2 spacing 11.54 along (0, 0, -1) of "Extrusion22"
sketch "Sketch4" plane through (-91.4015, 0, -67.7979) normal (-1, 0, 0) x (0, 0, 1)
  line L0 (0.0048, 0) -> (0.0048, 5) projected
  line L1 (0.0048, 0) -> (-0.9952, 0)
  line L2 (-0.9952, 0) -> (-0.9952, 1)
  line L3 (-0.9952, 1) -> (0.0048, 1)
  line L4 (0.0048, 1) -> (0.0048, 0)
  line L5 (9.6828, 0) -> (0.0048, 0) projected
  line L6 (9.6828, 0) -> (10.6828, 0)
  line L7 (10.6828, 0) -> (10.6828, 1)
  line L8 (10.6828, 1) -> (9.6828, 1)
  line L9 (9.6828, 1) -> (9.6828, 0)
  point P0 (67.7979, 0)
  dimension "d148" = 1
  dimension "d149" = 1
  dimension "d150" = 1
  dimension "d151" = 1
  constraints: 16 end point, 4 parallel, 2 horizontal, 2 perpendicular
  measures "d148" distance of L2.end L3.end
  measures "d149" distance of L1.end L2.end
  measures "d150" distance of L8.end L7.end
  measures "d151" distance of L7.end L6.end
extrude "Extrusion23" cut sketch "Sketch4" against normal blind 46
extrude "Extrusion24" add sketch "Sketch1" along normal blind 0.5 contours L33 L211 L273 L276 L275 L271 L35 L36 | L33 L207 L273 L209 | L269 L275 L267 L35 | L33 L203 L273 L205 | L265 L275 L263 L35 | L33 L199 L273 L201 | L261 L275 L259 L35 | L33 L195 L273 L197 | L257 L275 L255 L35 | L33 L191 L273 L193 | L253 L275 L251 L35 | L33 L187 L273 L189 | L249 L275 L247 L35 | L33 L183 L273 L185 | L245 L275 L243 L35 | L33 L179 L273 L181 | L241 L275 L239 L35 | L33 L175 L273 L177 | L237 L275 L235 L35 | L33 L171 L273 L173 | L233 L275 L231 L35 | L33 L167 L273 L169 | L229 L275 L227 L35 | L33 L163 L273 L165 | L225 L275 L223 L35 | L33 L159 L273 L161 | L221 L275 L219 L35 | L33 L154 L273 L157 | L217 L275 L215 L35 | L33 L34 L35 L213 L275 L274 L273 L156
sketch "Sketch5" plane through (0, 4, 0) normal (0, 1, 0) x (1, 0, 0)
  line L0 (-93.7167, 16.8415) -> (-91.8929, 16.8415)
  line L1 (-91.8929, 16.8415) -> (-91.8929, 18.5718)
  line L2 (-91.8929, 18.5718) -> (-93.7167, 18.5718)
  line L3 (-93.7167, 18.5718) -> (-93.7167, 16.8415)
  line L4 (-90.9167, 18.5718) -> (-90.9167, 16.8415)
  line L5 (-90.9167, 16.8415) -> (-89.0929, 16.8415)
  line L6 (-89.0929, 18.5718) -> (-90.9167, 18.5718)
  line L7 (-89.0929, 16.8415) -> (-89.0929, 18.5718)
  line L8 (-88.1167, 18.5718) -> (-88.1167, 16.8415)
  line L9 (-88.1167, 16.8415) -> (-86.2929, 16.8415)
  line L10 (-86.2929, 18.5718) -> (-88.1167, 18.5718)
  line L11 (-86.2929, 16.8415) -> (-86.2929, 18.5718)
  line L12 (-85.3167, 18.5718) -> (-85.3167, 16.8415)
  line L13 (-85.3167, 16.8415) -> (-83.4929, 16.8415)
  line L14 (-83.4929, 18.5718) -> (-85.3167, 18.5718)
  line L15 (-83.4929, 16.8415) -> (-83.4929, 18.5718)
  line L16 (-82.5167, 18.5718) -> (-82.5167, 16.8415)
  line L17 (-82.5167, 16.8415) -> (-80.6929, 16.8415)
  line L18 (-80.6929, 18.5718) -> (-82.5167, 18.5718)
  line L19 (-80.6929, 16.8415) -> (-80.6929, 18.5718)
  line L20 (-79.7167, 18.5718) -> (-79.7167, 16.8415)
  line L21 (-79.7167, 16.8415) -> (-77.8929, 16.8415)
  line L22 (-77.8929, 18.5718) -> (-79.7167, 18.5718)
  line L23 (-77.8929, 16.8415) -> (-77.8929, 18.5718)
  line L24 (-76.9167, 18.5718) -> (-76.9167, 16.8415)
  line L25 (-76.9167, 16.8415) -> (-75.0929, 16.8415)
  line L26 (-75.0929, 18.5718) -> (-76.9167, 18.5718)
  line L27 (-75.0929, 16.8415) -> (-75.0929, 18.5718)
  line L28 (-74.1167, 18.5718) -> (-74.1167, 16.8415)
  line L29 (-74.1167, 16.8415) -> (-72.2929, 16.8415)
  line L30 (-72.2929, 18.5718) -> (-74.1167, 18.5718)
  line L31 (-72.2929, 16.8415) -> (-72.2929, 18.5718)
  line L32 (-71.3167, 18.5718) -> (-71.3167, 16.8415)
  line L33 (-71.3167, 16.8415) -> (-69.4929, 16.8415)
  line L34 (-69.4929, 18.5718) -> (-71.3167, 18.5718)
  line L35 (-69.4929, 16.8415) -> (-69.4929, 18.5718)
  point P0 (0, 0)
  dimension "d158" = 2.8
  constraints: 72 end point, 2 horizontal, 2 parallel, 1 collinear, 1 perpendicular, 63 other
  measures "d158" distance of L2.end L4.start
extrude "Extrusion25" cut sketch "Sketch5" against normal blind 4
sketch "Sketch6" plane through (0, 4, 0) normal (0, 1, 0) x (1, 0, 0)
  line L0 (-63.7969, 16.492) -> (-62.6964, 16.492)
  line L1 (-62.6964, 16.492) -> (-62.6964, 18.493)
  line L2 (-62.6964, 18.493) -> (-63.7969, 18.493)
  line L3 (-63.7969, 18.493) -> (-63.7969, 16.492)
  point P0 (0, 0)
  constraints: 8 end point, 2 parallel, 1 horizontal, 1 perpendicular
extrude "Extrusion26" cut sketch "Sketch6" against normal blind 4
pattern_linear "Rectangular Pattern2" count 12 spacing 2.6 along (1, 0, 0) of "Extrusion26"
sketch "Sketch7" plane through (0, 4, 0) normal (0, 1, 0) x (1, 0, 0)
  line L0 (-93.0594, 79.9374) -> (-91.668, 79.9374)
  line L1 (-91.668, 79.9374) -> (-91.668, 81.9326)
  line L2 (-91.668, 81.9326) -> (-93.0594, 81.9326)
  line L3 (-93.0594, 81.9326) -> (-93.0594, 79.9374)
  point P0 (0, 0)
  constraints: 8 end point, 2 parallel, 1 horizontal, 1 perpendicular
extrude "Extrusion27" cut sketch "Sketch7" against normal blind 3.5
pattern_linear "Rectangular Pattern3" count 6 spacing 3.5 along (1, 0, 0) of "Extrusion27"
sketch "Sketch8" plane through (0, 4, 0) normal (0, 1, 0) x (1, 0, 0)
  line L0 (-70.1517, 80.4362) -> (-68.3317, 80.4362)
  line L1 (-68.3317, 80.4362) -> (-68.3317, 82.2567)
  line L2 (-68.3317, 82.2567) -> (-70.1517, 82.2567)
  line L3 (-70.1517, 82.2567) -> (-70.1517, 80.4362)
  point P0 (0, 0)
  dimension "d175" = 1.82
  constraints: 8 end point, 2 parallel, 1 horizontal, 1 perpendicular
  measures "d175" distance of L2.end L1.end
extrude "Extrusion28" cut sketch "Sketch8" against normal blind 3.5
pattern_linear "Rectangular Pattern4" count 7 spacing 3.8 along (1, 0, 0) of "Extrusion28"
fillet "Fillet5" radius 0.4 2 edges at (-29.24, 7, -72.0836) (-38.4488, 7, -72.0836)
decal "Decal1"
sketch "Sketch9" plane through (0, 0, 0) normal (0, 1, 0) x (1, 0, 0)
  circle A0 centre (-27.4955, 80.9948) radius 1.8325
  circle A1 centre (-29.6229, 18.3756) radius 1.8001
  circle A2 centre (-95.3983, 38.1049) radius 2.1773
  circle A3 centre (-95.3983, 74.4629) radius 1.6835
  point P0 (0, 0)
  constraints: 4 centre point
extrude "Extrusion29" cut sketch "Sketch9" against normal blind 3.5
scale "Scale1" factors (1.25, 1.25, 1.25) then translate (6.8739, 0.125, 20.2487) bodies 1
scale "Scale2" factors (0.94, 0.94, 0.94) then translate (-1.6497, -0.03, -4.8597) bodies 1
body "Solid1"
